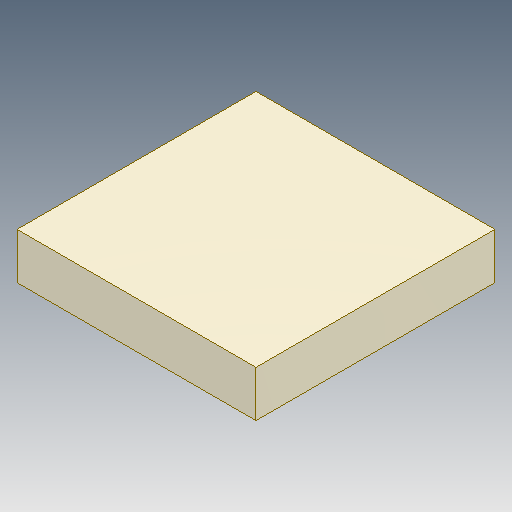
# Autodesk Inventor part: RESET
Saved by Autodesk Inventor 2017 (Build 210142000, 142)
## iProperties
Part Number: RESET
Material: Generisch
Document SubType Name: Modeling
Designer: Werkstatt
Density: 1 g/cm^3
Appearance: TACTILE_SWITCH_SMD, RESET
Author: Werkstatt
Autodesk Inventor part; units mm, degrees
ref_plane "YZ Plane" through (0, 0, 0) normal (1, 0, 0) x (0, 1, 0)
ref_plane "XZ Plane" through (0, 0, 0) normal (0, 1, 0) x (-1, 0, 0)
ref_plane "XY Plane" through (0, 0, 0) normal (0, 0, 1) x (1, 0, 0)
sketch "TACTILE_SWITCH_SMD, RESET_51" plane through (0, 0, 0) normal (0, 0, 1) x (1, 0, 0)
  line L0 (-2.6416, 2.54) -> (2.54, 2.54)
  line L1 (2.54, 2.54) -> (2.54, -2.6416)
  line L2 (2.54, -2.6416) -> (-2.6416, -2.6416)
  line L3 (-2.6416, -2.6416) -> (-2.6416, 2.54)
  constraints: 8 end point
extrude "Extrusion1" add sketch "TACTILE_SWITCH_SMD, RESET_51" along normal blind 1
